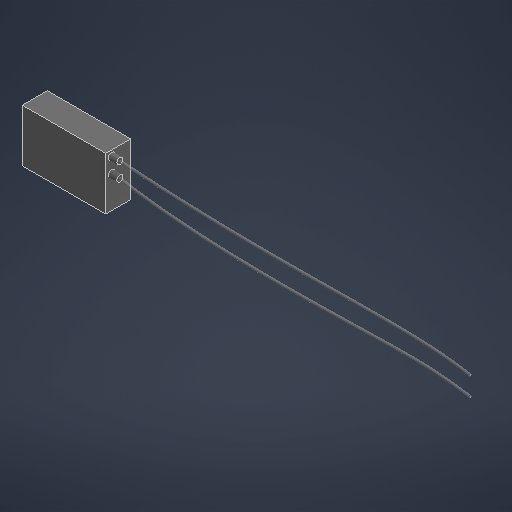
# Autodesk Inventor part: P_Receiver_Radiolink
Saved by Autodesk Inventor 2026 (Build 300175000, 175)
## iProperties
Created: 2025-08-28
Part Number: P_Receiver_Radiolink
Material: PET-Kunststoff
Document SubType Name: Modeling
Designer: FAL
Density: 1.541 g/cm^3
Appearance: Polycarbonat - klar
Author: FAL
Autodesk Inventor part; units mm, degrees
ref_plane "YZ Plane" through (0, 0, 0) normal (1, 0, 0) x (0, 1, 0)
ref_plane "XZ Plane" through (0, 0, 0) normal (0, 1, 0) x (-1, 0, 0)
ref_plane "XY Plane" through (0, 0, 0) normal (0, 0, 1) x (1, 0, 0)
sketch "Skizze1" plane through (0, 0, 0) normal (0, 1, 0) x (-1, 0, 0)
  line L0 (-25, 15.75) -> (25, 15.75)
  line L1 (25, 15.75) -> (25, -15.75)
  line L2 (25, -15.75) -> (-25, -15.75)
  line L3 (-25, -15.75) -> (-25, 15.75)
  line L4 (-25, 15.75) -> (25, -15.75) construction
  line L5 (25, 15.75) -> (-25, -15.75) construction
  point P0 (0, 0)
  dimension "d0" = 50
  dimension "d1" = 31.5
  constraints: 12 end point, 2 midpoint, 2 parallel, 1 horizontal, 1 perpendicular
  measures "d0" distance of L0.start L0.end
  measures "d1" distance of L0.end L1.end
extrude "Extrusion1" add sketch "Skizze1" along normal blind 15
sketch "Skizze2" plane through (25, 0, 15.75) normal (1, 0, 0) x (0, 0, -1)
  circle A0 centre (3.2281, 3.4997) radius 2
  circle A1 centre (12.2281, 3.4997) radius 2
  point P0 (15.75, 0)
  dimension "d4" = 4
  dimension "d5" = 9
  constraints: 2 centre point, 1 equal radius
  measures "d4" diameter of A1
  measures "d5" distance of A1.centre A0.centre
extrude "Extrusion2" add sketch "Skizze2" along normal blind 5 draft -2
sketch "Skizze3" plane through (30, 3.4997, 3.5219) normal (1, 0, 0) x (0, 0, -1)
  point P0 (3.5219, -3.4997)
sketch3d "3D-Skizze2"
ref_plane "Arbeitsebene1" through (36.5566, 3.4997, 12.5219) normal (0, 1, 0) x (0, 0, 1)
sketch "Skizze5" plane through (30, 3.4997, 12.5219) normal (1, 0, 0) x (0, 0, -1)
  circle A0 centre (0, 0) radius 0.75
  circle A1 centre (9, 0) radius 2 projected
  circle A2 centre (9, 0) radius 0.75
  circle A3 centre (0, 0) radius 1.8254 projected
  point P0 (12.5219, -3.4997)
  dimension "d11" = 1.5
  constraints: 2 centre point, 1 coincident, 1 concentric, 1 equal radius
  measures "d11" diameter of A2
sketch "Skizze4" plane through (36.5566, 3.4997, 12.5219) normal (0, 1, 0) x (0, 0, 1)
  line L0 (-1.8254, -6.5566) -> (1.8254, -6.5566) projected
  line L1 (0, -6.5566) -> (-7.608, 98.9489) construction
  line L2 (-7.608, 98.9489) -> (1.8254, 161.9077) construction
  line L3 (1.8254, 161.9077) -> (-6.2392, 203.4434) construction
  spline S0 degree 3 poles (0, -6.5566) (-7.608, 98.9489) (1.8254, 161.9077) (-6.2392, 203.4434) knots 1 1 1 1 2 2 2 2
  line L4 (-10.8254, -6.5566) -> (-7.1746, -6.5566) projected
  line L5 (-9, -6.5566) -> (-21.9877, 60.3348) construction
  line L6 (-21.9877, 60.3348) -> (-12.6894, 172.5713) construction
  line L7 (-12.6894, 172.5713) -> (-12.6894, 169.4169) construction
  line L8 (-12.6894, 169.4169) -> (-17.3386, 203.4434) construction
  spline S1 degree 4 poles (-9, -6.5566) (-21.9877, 60.3348) (-12.6894, 172.5713) (-12.6894, 169.4169) (-17.3386, 203.4434) knots 1 1 1 1 1 2 2 2 2 2
  point P0 (-12.5219, -36.5566)
  dimension "d10" = 210
  constraints: 2 midpoint, 1 perpendicular, 6 other
  measures "d10" distance from line of L0 L3.end
sweep "Sweeping1" add profiles "Skizze5" path "Skizze4" separate body path curves S0 contours A0
sweep "Sweeping2" add profiles "Skizze5" path "Skizze4" separate body path curves S1 contours A2
sketch "Skizze6" plane through (-25, 0, -15.75) normal (-1, 0, 0) x (0, 0, 1)
  line L0 (0.9623, 1.2562) -> (30.4832, 1.2562)
  line L1 (30.4832, 1.2562) -> (30.4832, 13.7162)
  line L2 (30.4832, 13.7162) -> (0.9623, 13.7162)
  line L3 (0.9623, 13.7162) -> (0.9623, 1.2562)
  point P0 (15.75, 0)
  constraints: 8 end point, 2 parallel, 1 horizontal, 1 perpendicular
extrude "Extrusion3" cut sketch "Skizze6" against normal blind 4.5 bodies 1
